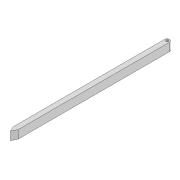
# Autodesk Inventor part: Part_10
Saved by Autodesk Inventor 2022 (Build 260153000, 153)
## iProperties
Created: 2022-05-03
Part Number: Part_10
Material: Generic
Document SubType Name: Modeling
Designer: dell
Density: 1 g/cm^3
Appearance: Default
Author: dell
Autodesk Inventor part; units mm, degrees
ref_plane "YZ Plane" through (0, 0, 0) normal (1, 0, 0) x (0, 1, 0)
ref_plane "XZ Plane" through (0, 0, 0) normal (0, 1, 0) x (-1, 0, 0)
ref_plane "XY Plane" through (0, 0, 0) normal (0, 0, 1) x (1, 0, 0)
sketch "Sketch1" plane through (0, 0, 0) normal (0, 1, 0) x (-1, 0, 0)
  line L0 (0, 0) -> (0, -441.93) construction
  line L1 (-3, 0) -> (-3, -441.93)
  line L2 (3, -441.93) -> (3, 0)
  arc A0 (3, 0) -> (-3, 0) centre (0, 0) ccw
  arc A1 (-3, -441.93) -> (3, -441.93) centre (0, -441.93) ccw
  circle A2 centre (0, 0) radius 1.5
  circle A3 centre (0, -441.93) radius 1.5
  circle A4 centre (0, -48.203) radius 1.5
  circle A5 centre (0, -166.766) radius 1.5
  arc A6 (-3, -163.766) -> (-3, -51.203) centre (-399.0207, -107.4845) ccw
  arc A7 (3, -163.766) -> (3, -51.203) centre (-393.0207, -107.4845) ccw
  point P0 (0, -220.965)
  dimension "d0" = 6
  dimension "d1" = 441.93
  dimension "d2" = 3
  dimension "d3" = 3
  dimension "d20" = 3
  dimension "d21" = 48.203
  dimension "d22" = 3
  dimension "d23" = 166.766
  dimension "d24" = 400
  dimension "d25" = 400
  dimension "d26" = 3
  dimension "d28" = 3
  constraints: 8 centre point, 8 end point, 8 point on circle, 6 point on line, 4 tangent, 2 coincident, 2 horizontal alignment, 1 midpoint, 1 parallel, 1 vertical
  measures "d0" diameter of A1
  measures "d1" distance of L0.end L0.start
  measures "d2" diameter of A2
  measures "d3" diameter of A3
  measures "d20" diameter of A4
  measures "d21" distance of L0.start A4.centre
  measures "d22" diameter of A5
  measures "d23" distance of L0.start A5.centre
  measures "d24" radius of A6
  measures "d25" radius of A7
  measures "d26" horizontal distance of A5.centre A6.start
  measures "d28" horizontal distance of A4.centre A6.end
extrude "Extrusion1" add sketch "Sketch1" along normal blind 10 contours A0 L2 A1 L1 A6 | A7 L2
sketch "Sketch2" plane through (0, 10, 0) normal (0, 1, 0) x (1, 0, 0)
  line L0 (3, 0) -> (3, 51.203) projected
  arc A0 (3, 163.766) -> (3, 51.203) centre (399.0207, 107.4845) ccw projected
  line L1 (3, 163.766) -> (3, 441.93) projected
  arc A1 (3, 441.93) -> (-3, 441.93) centre (0, 441.93) ccw projected
  line L2 (-3, 441.93) -> (-3, 163.766) projected
  arc A2 (-3, 163.766) -> (-3, 51.203) centre (393.0207, 107.4845) ccw projected
  line L3 (-3, 51.203) -> (-3, 0) projected
  arc A3 (-3, 0) -> (3, 0) centre (0, 0) ccw projected
  circle A4 centre (0, 0) radius 1.5 projected
  circle A5 centre (0, 441.93) radius 1.5 projected
  circle A6 centre (0, 166.766) radius 1.5 projected
  circle A7 centre (0, 48.203) radius 1.5 projected
  line L4 (-3, 258.3394) -> (0, 251.9059)
  line L5 (0, 251.9059) -> (3, 258.3394)
  dimension "d29" = 25
  dimension "d30" = 25
  constraints: 4 end point, 2 point on line
  measures "d29" angle of L2 L4
  measures "d30" angle of L1 L5
extrude "Extrusion2" cut sketch "Sketch2" against normal blind 100 contours A3 L3 A2 L2 L4 L5 L1 A0 L0
body "Solid1"
